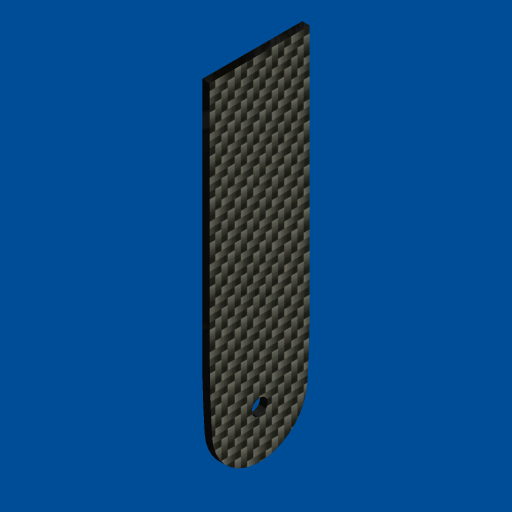
# Autodesk Inventor part: wristPlate
Saved by Autodesk Inventor 2023 (Build 270158030, 158C)
## iProperties
Created: 2023-03-03
Part Number: wristPlate
Material: Generic
Document SubType Name: Modeling
Designer: kumpu
Density: 1 g/cm^3
Appearance: Glossy - Black
Author: kumpu
Autodesk Inventor part; units mm, degrees
ref_plane "YZ Plane" through (0, 0, 0) normal (1, 0, 0) x (0, 1, 0)
ref_plane "XZ Plane" through (0, 0, 0) normal (0, 1, 0) x (-1, 0, 0)
ref_plane "XY Plane" through (0, 0, 0) normal (0, 0, 1) x (1, 0, 0)
sketch "Sketch1" plane through (0, 0, 0) normal (1, 0, 0) x (0, 1, 0)
  line L0 (122, 20) -> (28, 20)
  arc A0 (28, 20) -> (-1.2912, 19.0062) centre (28, -412.1566) ccw
  arc A1 (-1.2912, 19.0062) -> (-19.05, 0) centre (0, 0) ccw
  line L1 (-19.05, 0) -> (122, 0)
  line L2 (122, 0) -> (122, 20)
  circle A2 centre (0, 0) radius 3.175
  point P0 (-3.175, 0)
  point P1 (3.175, 0)
  dimension "d0" = 19.05
  dimension "d1" = 6.35
  dimension "d2" = 122
  dimension "d3" = 94
  dimension "d4" = 20
  constraints: 6 end point, 4 point on circle, 3 centre point, 2 coincident, 2 horizontal, 2 tangent, 1 perpendicular, 1 point on line
  measures "d0" radius of A1
  measures "d1" diameter of A2
  measures "d2" distance from line of point (0, 0) L2
  measures "d3" distance of L0.start L0.end
  measures "d4" distance of L1.end L0.start
extrude "Extrusion1" add sketch "Sketch1" along normal blind 3 contours L2 L1 A2 A1 A0 L0
mirror "Mirror1" about plane through (0, 0, 0) normal (0, 0, 1) of "Extrusion1"
body "Solid1"
